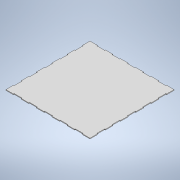
# Autodesk Inventor part: base
Saved by Autodesk Inventor 2020 (Build 240168000, 168)
## iProperties
Created: 2020-03-06
Part Number: base
Material: Generic
Document SubType Name: Modeling
Designer: udvarhelyi
Density: 1 g/cm^3
Appearance: Default
Author: udvarhelyi
Autodesk Inventor part; units mm, degrees
ref_plane "YZ Plane" through (0, 0, 0) normal (1, 0, 0) x (0, 1, 0)
ref_plane "XZ Plane" through (0, 0, 0) normal (0, 1, 0) x (-1, 0, 0)
ref_plane "XY Plane" through (0, 0, 0) normal (0, 0, 1) x (1, 0, 0)
sketch "Sketch1" plane through (0, 0, 0) normal (0, 1, 0) x (-1, 0, 0)
  line L0 (143.1818, 175) -> (143.1818, 172)
  line L1 (111.3636, 172) -> (111.3636, 175)
  line L2 (79.5455, 175) -> (79.5455, 172)
  line L3 (47.7273, 172) -> (47.7273, 175)
  line L4 (15.9091, 175) -> (15.9091, 172)
  line L5 (-15.9091, 172) -> (-15.9091, 175)
  line L6 (-47.7273, 175) -> (-47.7273, 172)
  line L7 (-79.5455, 172) -> (-79.5455, 175)
  line L8 (-111.3636, 175) -> (-111.3636, 172)
  line L9 (-143.1818, 172) -> (-143.1818, 175)
  line L10 (-175, 143.1818) -> (-172, 143.1818)
  line L11 (-172, 111.3636) -> (-175, 111.3636)
  line L12 (-175, 79.5455) -> (-172, 79.5455)
  line L13 (-172, 47.7273) -> (-175, 47.7273)
  line L14 (-175, 15.9091) -> (-172, 15.9091)
  line L15 (-172, -15.9091) -> (-175, -15.9091)
  line L16 (-172, -47.7273) -> (-175, -47.7273)
  line L17 (-175, -79.5455) -> (-172, -79.5455)
  line L18 (-172, -111.3636) -> (-175, -111.3636)
  line L19 (-175, -143.1818) -> (-172, -143.1818)
  line L20 (-143.1818, -175) -> (-143.1818, -172)
  line L21 (-111.3636, -172) -> (-111.3636, -175)
  line L22 (-79.5455, -175) -> (-79.5455, -172)
  line L23 (-47.7273, -172) -> (-47.7273, -175)
  line L24 (-15.9091, -172) -> (-15.9091, -175)
  line L25 (15.9091, -175) -> (15.9091, -172)
  line L26 (143.1818, -172) -> (143.1818, -175)
  line L27 (111.3636, -175) -> (111.3636, -172)
  line L28 (79.5455, -172) -> (79.5455, -175)
  line L29 (47.7273, -175) -> (47.7273, -172)
  line L30 (172, -143.1818) -> (175, -143.1818)
  line L31 (175, -111.3636) -> (172, -111.3636)
  line L32 (175, -79.5455) -> (172, -79.5455)
  line L33 (175, -15.9091) -> (172, -15.9091)
  line L34 (175, 15.9091) -> (172, 15.9091)
  line L35 (175, 143.1818) -> (172, 143.1818)
  line L36 (172, 111.3636) -> (175, 111.3636)
  line L37 (175, 79.5455) -> (172, 79.5455)
  line L38 (172, 47.7273) -> (175, 47.7273)
  line L39 (111.3636, -172) -> (143.1818, -172)
  line L40 (47.7273, -172) -> (79.5455, -172)
  line L41 (-15.9091, -172) -> (15.9091, -172)
  line L42 (172, -143.1818) -> (172, -111.3636)
  line L43 (172, -15.9091) -> (172, 15.9091)
  line L44 (172, 47.7273) -> (172, 79.5455)
  line L45 (172, 111.3636) -> (172, 143.1818)
  line L46 (143.1818, 172) -> (111.3636, 172)
  line L47 (79.5455, 172) -> (47.7273, 172)
  line L48 (15.9091, 172) -> (-15.9091, 172)
  line L49 (-47.7273, 172) -> (-79.5455, 172)
  line L50 (-111.3636, 172) -> (-143.1818, 172)
  line L51 (-172, 143.1818) -> (-172, 111.3636)
  line L52 (-172, 79.5455) -> (-172, 47.7273)
  line L53 (-172, 15.9091) -> (-172, -15.9091)
  line L54 (-175, 47.7273) -> (-175, 15.9091)
  line L55 (-175, 175) -> (-175, 143.1818)
  line L56 (-175, 111.3636) -> (-175, 79.5455)
  line L57 (-143.1818, -172) -> (-111.3636, -172)
  line L58 (-79.5455, -172) -> (-47.7273, -172)
  line L59 (-172, -47.7273) -> (-172, -79.5455)
  line L60 (-172, -111.3636) -> (-172, -143.1818)
  line L61 (-175, -15.9091) -> (-175, -47.7273)
  line L62 (-175, -79.5455) -> (-175, -111.3636)
  line L63 (-175, -143.1818) -> (-175, -175)
  line L64 (-175, -175) -> (-143.1818, -175)
  line L65 (-111.3636, -175) -> (-79.5455, -175)
  line L66 (-47.7273, -175) -> (-15.9091, -175)
  line L67 (15.9091, -175) -> (47.7273, -175)
  line L68 (79.5455, -175) -> (111.3636, -175)
  line L69 (143.1818, -175) -> (175, -175)
  line L70 (175, -175) -> (175, -143.1818)
  line L71 (175, 15.9091) -> (175, 47.7273)
  line L72 (175, 79.5455) -> (175, 111.3636)
  line L73 (175, 143.1818) -> (175, 175)
  line L74 (175, 175) -> (143.1818, 175)
  line L75 (111.3636, 175) -> (79.5455, 175)
  line L76 (47.7273, 175) -> (15.9091, 175)
  line L77 (-15.9091, 175) -> (-47.7273, 175)
  line L78 (-79.5455, 175) -> (-111.3636, 175)
  line L79 (-143.1818, 175) -> (-175, 175)
  line L80 (172, -79.5455) -> (172, -47.7273)
  line L81 (172, -47.7273) -> (175, -47.7273)
  line L82 (175, -111.3636) -> (175, -79.5455)
  line L83 (175, -47.7273) -> (175, -15.9091)
  point P0 (0, 0)
  dimension "d1" = 350
  dimension "d3" = 350
  dimension "d5" = 175
  dimension "d6" = 175
  dimension "d7" = 3
  dimension "d8" = 3
  dimension "d9" = 3
  dimension "d10" = 3
  constraints: 249 perpendicular, 168 end point, 121 parallel, 56 collinear, 20 equal length, 6 horizontal, 1 vertical
  measures "d1" distance of L63.end L69.end
  measures "d3" distance of L69.end L73.end
  measures "d5" horizontal distance of L69.end point (0, 0)
  measures "d6" horizontal distance of L69.end point (0, 0)
  measures "d7" distance of L26.start L26.end
  measures "d8" distance of L30.start L30.end
  measures "d9" distance of L19.start L19.end
  measures "d10" distance of L9.start L9.end
extrude "Extrusion1" add sketch "Sketch1" along normal blind 3
equation "\"d1\" = wt"
equation "\"d3\" = lt"
equation "\"d5\" = 0.5 * lt"
equation "\"d6\" = 0.5 * wt"
equation "\"d7\" = tt"
equation "\"d8\" = tt"
equation "\"d9\" = tt"
equation "\"d10\" = tt"
equation "\"d13\" = tt"
equation "\"wt\" = 350"
equation "\"tt\" = 3"
equation "\"tol\" = 0"
equation "\"tiroir\" = 25.4"
equation "\"nHoles\" = 101.6"
equation "\"shelfH\" = 35"
equation "\"d0\" = 0.5 * wt"
equation "\"d2\" = 0.5 * lt"
equation "\"lt\" = 350"
equation "\"d4\" = tt"
body "Solid1"
